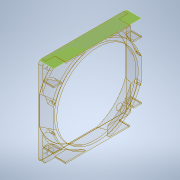
# Autodesk Inventor part: Surface 5
Saved by Autodesk Inventor 2022.1 (Build 261234000, 234)
## iProperties
Created: 2021-08-19
Part Number: Surface 5
Material: PC/ABS Plastic
Document SubType Name: Modeling
Designer: robst
Density: 0.357273 g/cm^3
Appearance: Olive Green
Author: robst
Autodesk Inventor part; units mm, degrees
ref_plane "YZ Plane" through (0, 0, 0) normal (1, 0, 0) x (0, 1, 0)
ref_plane "XZ Plane" through (0, 0, 0) normal (0, 1, 0) x (-1, 0, 0)
ref_plane "XY Plane" through (0, 0, 0) normal (0, 0, 1) x (1, 0, 0)
surface "Composite1"
sketch "Sketch1" plane through (-100, 253.7713, 21.8) normal (0, 1, 0) x (1, 0, 0)
  line L0 (-10.1736, 51.8) -> (-10.1736, 49.7) projected
  line L1 (0, -8.1) -> (0, -2.8) projected
  line L2 (-10.1736, 51.8) -> (0, 51.8)
  line L3 (0, 51.8) -> (0, -8.1)
  line L4 (0, -8.1) -> (-10.1736, -8.1)
  line L5 (-10.1736, -8.1) -> (-10.1736, 51.8)
  point P0 (100, 21.8)
  constraints: 8 end point, 2 parallel, 1 horizontal, 1 perpendicular
extrude "Extrusion1" add sketch "Sketch1" against normal blind 0.1
body "Solid1"
body "Srf1"
